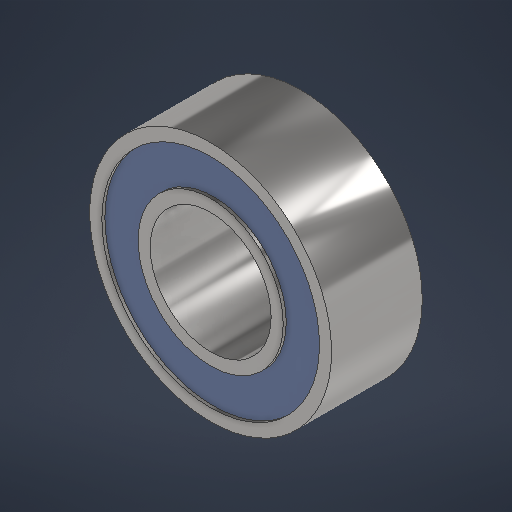
# Autodesk Inventor part: Kugellager 8 x 4 x 3
Saved by Autodesk Inventor 2025.2 (Build 292293000, 293)
## iProperties
Created: 2024-11-27
Part Number: Kugellager 8 x 4 x 3
Material: Generisch
Document SubType Name: Modeling
Designer: Fabian
Density: 1 g/cm^3
Appearance: Vorgabe
Author: Fabian
Autodesk Inventor part; units mm, degrees
ref_plane "YZ Plane" through (0, 0, 0) normal (1, 0, 0) x (0, 1, 0)
ref_plane "XZ Plane" through (0, 0, 0) normal (0, 1, 0) x (-1, 0, 0)
ref_plane "XY Plane" through (0, 0, 0) normal (0, 0, 1) x (1, 0, 0)
sketch "Skizze1" plane through (0, 0, 0) normal (0, 0, 1) x (1, 0, 0)
  circle A0 centre (0, 0) radius 2
  circle A1 centre (0, 0) radius 4
  circle A2 centre (0, 0) radius 2.4
  circle A3 centre (0, 0) radius 3.6
  dimension "d0" = 4
  dimension "d1" = 8
  dimension "d3" = 0.4
  dimension "d4" = 0.4
  constraints: 4 centre point, 4 coincident
  measures "d0" diameter of A0
  measures "d1" diameter of A1
  measures "d3" radial gap between concentric circles of A3 A1
  measures "d4" radial gap between concentric circles of A0 A2
extrude "Extrusion1" add sketch "Skizze1" along normal mid plane 2.8 contours A3
extrude "Extrusion2" add sketch "Skizze1" along normal mid plane 3
